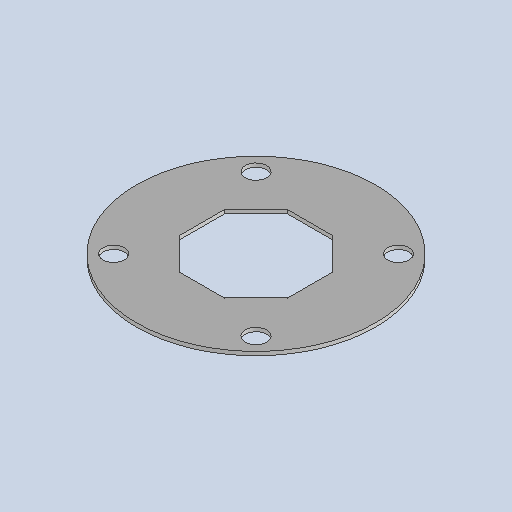
# Autodesk Inventor part: PRS 1651 FDS MAIN  FLANGE_940
Saved by Autodesk Inventor 2026.2 (Build 302298000, 298)
## iProperties
Created: 2025-06-24
Part Number: PRS 1651 FDS MAIN  FLANGE_940
Material: Stainless Steel
Document SubType Name: Sheet Metal
Designer: admin
Mass: 326.359 g
Surface Area: 301.648 cm^2
Volume: 40.7948 cm^3
Density: 8 g/cm^3
Flat Pattern Width: 19 cm
Flat Pattern Length: 19 cm
Flat Pattern Area: 361 cm^2
Sheet Metal Rule: Default
Sheet Metal Width: 190,000 mm
Sheet Metal Length: 190,000 mm
Sheet Metal Area: 36100,000 mm^2
Appearance: Default
Author: user
Autodesk Inventor part; units mm, degrees
ref_plane "YZ Plane" through (0, 0, 0) normal (1, 0, 0) x (0, 1, 0)
ref_plane "XZ Plane" through (0, 0, 0) normal (0, 1, 0) x (-1, 0, 0)
ref_plane "XY Plane" through (0, 0, 0) normal (0, 0, 1) x (1, 0, 0)
sketch "Sketch1" plane through (0, 0, 0) normal (0, 0, 1) x (1, 0, 0)
  circle A0 centre (0, 0) radius 95
  circle A1 centre (-56.5685, 56.5685) radius 8.5
  circle A2 centre (0, 0) radius 80 construction
  circle A3 centre (-56.5685, -56.5685) radius 8.5
  circle A4 centre (56.5685, -56.5685) radius 8.5
  circle A5 centre (56.5685, 56.5685) radius 8.5
  line L0 (17.8112, -43) -> (-17.8112, -43)
  line L1 (-17.8112, -43) -> (-43, -17.8112)
  line L2 (-43, -17.8112) -> (-43, 17.8112)
  line L3 (-43, 17.8112) -> (-17.8112, 43)
  line L4 (-17.8112, 43) -> (17.8112, 43)
  line L5 (17.8112, 43) -> (43, 17.8112)
  line L6 (43, 17.8112) -> (43, -17.8112)
  line L7 (43, -17.8112) -> (17.8112, -43)
  line L8 (0, 0) -> (-30.4056, 30.4056) construction
  dimension "d171" = 160
  dimension "d157" = 190
  dimension "d170" = 17
  dimension "d174" = 360
  dimension "d176" = 86
  measures "d157" diameter of A0
  measures "d170" diameter of A1
  measures "d176" distance between parallel lines of L4 L0
extrude "Plate5" add sketch "Sketch1" along normal blind 3
body "Solid3"
